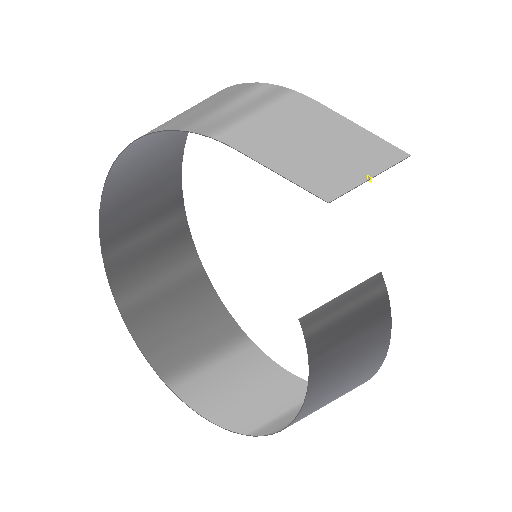
# Autodesk Inventor part: band
Saved by Autodesk Inventor 2022 (Build 260148000, 148)
## iProperties
Created: 2007-05-11
Part Number: band
Material: Steel, Mild
Document SubType Name: Sheet Metal
Designer: LionelF
Density: 7.86 g/cm^3
Mass: 40965.5 g
Surface Area: 33092.1 cm^2
Volume: 5211.9 cm^3
Sheet Metal Rule: Default
Appearance: Steel
Author: LionelF
Autodesk Inventor part; units mm, degrees
note: some values were not read from the file. Left out: dimensions or parameters whose unit could not be read.
ref_plane "YZ Plane" through (0, 0, 0) normal (1, 0, 0) x (0, 1, 0)
ref_plane "XZ Plane" through (0, 0, 0) normal (0, 1, 0) x (-1, 0, 0)
ref_plane "XY Plane" through (0, 0, 0) normal (0, 0, 1) x (1, 0, 0)
sketch "Sketch1" plane through (0, 0, 0) normal (0, 0, 1) x (1, 0, 0)
  circle A0 centre (15.9889, 3.0332) radius 69.85 construction
  line L0 (85.8389, 3.0332) -> (50.9139, -57.4587) construction
  line L1 (50.9139, -57.4587) -> (-18.9361, -57.4587) construction
  line L2 (-18.9361, -57.4587) -> (-53.8611, 3.0332) construction
  line L3 (-53.8611, 3.0332) -> (-18.9361, 63.5251) construction
  line L4 (-18.9361, 63.5251) -> (50.9139, 63.5251) construction
  line L5 (50.9139, 63.5251) -> (85.8389, 3.0332) construction
  line L6 (85.8389, 3.0332) -> (85.8389, 780.9082) construction
  line L7 (85.8389, 3.0332) -> (85.8389, 3.0332) construction
  line L8 (-53.8611, 3.0332) -> (85.8389, 3.0332) construction
  arc A1 (85.8389, 780.9082) -> (-303.0986, 676.6927) centre (85.8389, 3.0332) ccw
  arc A2 (-303.0986, 676.6927) -> (-657.1111, 63.5251) centre (50.9139, 63.5251) ccw
  arc A3 (-657.1111, 63.5251) -> (-338.0236, -489.1507) centre (-18.9361, 63.5251) ccw
  arc A4 (-338.0236, -489.1507) -> (230.3014, -489.1507) centre (-53.8611, 3.0332) ccw
  arc A5 (230.3014, -489.1507) -> (479.5389, -57.4587) centre (-18.9361, -57.4587) ccw
  line L9 (85.8389, 780.9082) -> (587.4889, 780.9082)
  circle A6 centre (435.5017, 175.6262) radius 21.082 construction
  line L10 (50.9139, -57.4587) -> (435.5017, 175.6262) construction
  line L11 (85.8389, 784.0832) -> (587.4889, 784.0832)
  arc A7 (85.8389, 784.0832) -> (-304.6861, 679.4423) centre (85.8389, 3.0332) ccw
  arc A8 (-304.6861, 679.4423) -> (-660.2861, 63.5251) centre (50.9139, 63.5251) ccw
  arc A9 (-660.2861, 63.5251) -> (-339.6111, -491.9003) centre (-18.9361, 63.5251) ccw
  arc A10 (-339.6111, -491.9003) -> (231.8889, -491.9003) centre (-53.8611, 3.0332) ccw
  arc A11 (231.8889, -491.9003) -> (482.7139, -57.4587) centre (-18.9361, -57.4587) ccw
  line L12 (587.4889, 784.0832) -> (587.4889, 780.9082)
  line L13 (15.9889, 72.8832) -> (15.9889, -66.8168) construction
  line L14 (425.7203, 156.9507) -> (423.0042, 155.3045)
  arc A12 (482.7139, -57.4587) -> (425.7203, 156.9507) centre (50.9139, -57.4587) ccw
  arc A13 (479.5389, -57.4587) -> (423.0042, 155.3045) centre (50.9139, -57.4587) ccw
  arc A14 (423.0042, 155.3045) -> (417.4725, 164.6993) centre (50.9139, -57.4587) ccw construction
  dimension "d2" = 42.164
  dimension "d1" = 777.875
  dimension "d3" = 172.593
  dimension "d5" = 449.707
  dimension "d6" = 3.175
  dimension "d8" = 571.5
  dimension "d9" = 428.625
  constraints: 30 end point, 30 point on circle, 14 centre point, 8 coincident, 8 tangent, 4 parallel, 3 perpendicular, 1 collinear, 1 midpoint, 1 point on line, 18 other
  measures "d1" distance of L0.start L6.end
  measures "d3" distance from line of L8 L10.end
  measures "d5" distance of L10.start L10.end
  measures "d6" distance of L11.end L9.end
  measures "d8" distance between parallel lines of L12 L13
  measures "d9" radius of A13
extrude "Extrusion1" add sketch "Sketch1" along normal blind 447.675
ref_plane "Work Plane1" through (587.4889, 784.0832, 223.8375) normal (0, 0, 1) x (1, 0, 0)
equation "\"d5\" = d4 + 0.5 * d2"
equation "\"BendRadius\" = Thickness"
equation "\"BendReliefWidth\" = Thickness"
equation "\"BendReliefDepth\" = 0.5 * Thickness"
equation "\"CornerReliefSize\" = 4 * Thickness"
equation "\"MinimumRemnant\" = 2 * Thickness"
equation "\"TransitionRadius\" = BendRadius"
equation "\"JacobiRadiusSize\" = Thickness"
equation "\"GapSize\" = Thickness"
equation "\"d4\" = 428.625"
equation "\"Thickness\" = 3.175"
body "Solid1"
